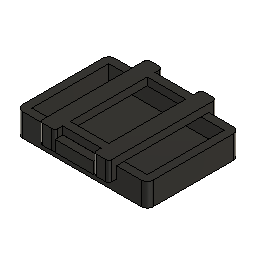
IRreceiverMount (Autodesk Fusion 360 design; units mm, degrees)
Autodesk Fusion 360 part; units mm, degrees
sketch "Sketch1" plane through (0, 0, 0) normal (0, 0, 1) x (1, 0, 0)
  line L0 (0, 0) -> (23.8125, 0)
  line L1 (23.8125, 0) -> (23.8125, 15.875)
  line L2 (23.8125, 15.875) -> (0, 15.875)
  line L3 (0, 15.875) -> (0, 0)
  line L4 (-0.3175, -1.5875) -> (24.13, -1.5875)
  line L5 (25.4, -0.3175) -> (25.4, 16.1925)
  line L6 (24.13, 17.4625) -> (-0.3175, 17.4625)
  line L7 (-1.5875, 16.1925) -> (-1.5875, -0.3175)
  arc A0 (-0.3175, 17.4625) -> (-1.5875, 16.1925) centre (-0.3175, 16.1925) ccw
  arc A1 (-1.5875, -0.3175) -> (-0.3175, -1.5875) centre (-0.3175, -0.3175) ccw
  arc A2 (25.4, 16.1925) -> (24.13, 17.4625) centre (24.13, 16.1925) ccw
  arc A3 (24.13, -1.5875) -> (25.4, -0.3175) centre (24.13, -0.3175) ccw
  dimension "d1" = 23.8125
  dimension "d2" = 15.875
  dimension "d4" = 1.27
  constraint coincident L0.start L3.end
  constraint horizontal L0
  constraint perpendicular L0 L1
  constraint perpendicular L1 L2
  constraint perpendicular L0 L3
  constraint tangent L6 A0
  constraint tangent L7 A0
  constraint tangent L4 A1
  constraint tangent L7 A1
  constraint equal A0 A1
  constraint tangent L5 A2
  constraint tangent L6 A2
  constraint equal A0 A2
  constraint tangent L4 A3
  constraint tangent L5 A3
  constraint equal A0 A3
  measures "d1" distance of L0.start L0.end
  measures "d2" distance of L0.end L1.end
  measures "d4" radius of A0
extrude "Extrude1" add sketch "Sketch1" along normal blind 1.5875 contours L0 L1 L2 L3 makes body 1
extrude "Extrude2" add sketch "Sketch1" along normal blind 4.7625 bodies 1
sketch "Sketch2" plane through (0, 0, 4.7625) normal (0, 0, 1) x (-1, 0, 0)
  line L0 (0, 0) -> (0, -15.875)
  line L1 (0, -15.875) -> (-23.8125, -15.875)
  line L2 (-23.8125, -15.875) -> (-23.8125, 0)
  line L3 (-23.8125, 0) -> (0, 0)
  arc A0 (-24.13, 1.5875) -> (-25.4, 0.3175) centre (-24.13, 0.3175) ccw
  line L4 (-25.4, 0.3175) -> (-25.4, -16.1925)
  arc A1 (-25.4, -16.1925) -> (-24.13, -17.4625) centre (-24.13, -16.1925) ccw
  line L5 (-24.13, -17.4625) -> (0.3175, -17.4625)
  arc A2 (0.3175, -17.4625) -> (1.5875, -16.1925) centre (0.3175, -16.1925) ccw
  line L6 (1.5875, -16.1925) -> (1.5875, 0.3175)
  arc A3 (1.5875, 0.3175) -> (0.3175, 1.5875) centre (0.3175, 0.3175) ccw
  line L7 (0.3175, 1.5875) -> (-24.13, 1.5875)
  line L8 (1.5875, -7.9375) -> (-25.4, -7.9375)
  line L9 (1.5875, -7.9375) -> (-4.7625, -7.9375)
  line L10 (-4.7625, -7.9375) -> (-7.9375, -7.9375)
  line L11 (-25.4, -7.9375) -> (-19.05, -7.9375)
  line L12 (-19.05, -7.9375) -> (-15.875, -7.9375)
  line L13 (-7.9375, -7.9375) -> (-7.9375, 1.5875)
  line L14 (-7.9375, -7.9375) -> (-7.9375, -17.4625)
  line L15 (-7.9375, -17.4625) -> (-4.7625, -17.4625)
  line L16 (-4.7625, -17.4625) -> (-4.7625, 1.5875)
  line L17 (-4.7625, 1.5875) -> (-7.9375, 1.5875)
  line L18 (-15.875, -7.9375) -> (-15.875, -17.4625)
  line L19 (-19.05, -7.9375) -> (-19.05, -17.4625)
  line L20 (-15.875, -17.4625) -> (-19.05, -17.4625)
  line L21 (-19.05, -7.9375) -> (-19.05, 1.5875)
  line L22 (-19.05, 1.5875) -> (-15.875, 1.5875)
  line L23 (-15.875, -7.9375) -> (-15.875, 1.5875)
  line L24 (-7.9375, -15.875) -> (-15.875, -15.875)
  line L25 (-15.875, -17.4625) -> (-7.9375, -17.4625)
  line L26 (-7.9375, 1.5875) -> (-15.875, 1.5875)
  line L27 (-15.875, 0) -> (-7.9375, 0)
  line L28 (-4.7625, 1.5875) -> (-4.7625, 2.54)
  line L29 (-5.3975, 3.175) -> (-7.3025, 3.175)
  line L30 (-7.9375, 2.54) -> (-7.9375, 1.5875)
  line L31 (-15.875, 1.5875) -> (-15.875, 2.54)
  line L32 (-16.51, 3.175) -> (-18.415, 3.175)
  line L33 (-19.05, 2.54) -> (-19.05, 1.5875)
  line L34 (-19.05, -17.4625) -> (-19.05, -18.415)
  line L35 (-18.415, -19.05) -> (-16.51, -19.05)
  line L36 (-15.875, -18.415) -> (-15.875, -17.4625)
  line L37 (-7.9375, -17.4625) -> (-7.9375, -18.415)
  line L38 (-7.3025, -19.05) -> (-5.3975, -19.05)
  line L39 (-4.7625, -18.415) -> (-4.7625, -17.4625)
  arc A4 (-5.3975, -19.05) -> (-4.7625, -18.415) centre (-5.3975, -18.415) ccw
  arc A5 (-7.9375, -18.415) -> (-7.3025, -19.05) centre (-7.3025, -18.415) ccw
  arc A6 (-16.51, -19.05) -> (-15.875, -18.415) centre (-16.51, -18.415) ccw
  arc A7 (-19.05, -18.415) -> (-18.415, -19.05) centre (-18.415, -18.415) ccw
  arc A8 (-4.7625, 2.54) -> (-5.3975, 3.175) centre (-5.3975, 2.54) ccw
  arc A9 (-7.3025, 3.175) -> (-7.9375, 2.54) centre (-7.3025, 2.54) ccw
  arc A10 (-15.875, 2.54) -> (-16.51, 3.175) centre (-16.51, 2.54) ccw
  arc A11 (-18.415, 3.175) -> (-19.05, 2.54) centre (-18.415, 2.54) ccw
  line L40 (-6.35, 1.5875) -> (-6.35, 1.6129)
  line L41 (-6.35, 1.6129) -> (-7.9375, 1.6129)
  line L42 (-6.35, 1.6129) -> (-4.7625, 1.6129)
  line L43 (-17.4625, 1.5875) -> (-17.4625, 1.6129)
  line L44 (-17.4625, 1.6129) -> (-19.05, 1.6129)
  line L45 (-17.4625, 1.6129) -> (-15.875, 1.6129)
  line L46 (-17.4625, -17.4625) -> (-17.4625, -17.4879)
  line L47 (-17.4625, -17.4879) -> (-19.05, -17.4879)
  line L48 (-17.4625, -17.4879) -> (-15.875, -17.4879)
  line L49 (-6.35, -17.4625) -> (-6.35, -17.4879)
  line L50 (-6.35, -17.4879) -> (-7.9375, -17.4879)
  line L51 (-6.35, -17.4879) -> (-4.7625, -17.4879)
  point P0 (-4.7625, 3.175)
  point P1 (-15.875, 3.175)
  point P2 (-19.05, -19.05)
  point P3 (-7.9375, -19.05)
  dimension "d9" = 6.35
  dimension "d10" = 3.175
  dimension "d11" = 6.35
  dimension "d12" = 3.175
  dimension "d13" = 3.175
  dimension "d14" = 3.175
  dimension "d15" = 1.5875
  dimension "d16" = 1.5875
  dimension "d17" = 1.5875
  dimension "d18" = 1.5875
  dimension "d19" = 0.635
  dimension "d22" = 0.0254
  dimension "d23" = 0.0254
  dimension "d24" = 0.0254
  dimension "d25" = 0.0254
  constraint midpoint L6 L8.start
  constraint midpoint L4 L8.end
  constraint coincident L8 L9.end
  constraint perpendicular L0 L10
  constraint perpendicular L2 L11
  constraint perpendicular L2 L12
  constraint coincident L7 L13.end
  constraint perpendicular L7 L13
  constraint coincident L5 L14.end
  constraint perpendicular L5 L14
  constraint coincident L5 L15.end
  constraint coincident L7 L16.end
  constraint perpendicular L7 L16
  constraint coincident L5 L18.end
  constraint perpendicular L5 L18
  constraint coincident L5 L19.end
  constraint perpendicular L5 L19
  constraint coincident L7 L21.end
  constraint perpendicular L7 L21
  constraint coincident L7 L22.end
  constraint coincident L14 L24.start
  constraint coincident L1 L24.start
  constraint coincident L18 L24.end
  constraint coincident L1 L24.end
  constraint coincident L23 L27.start
  constraint coincident L3 L27.start
  constraint coincident L13 L27.end
  constraint coincident L3 L27.end
  constraint perpendicular L17 L28
  constraint perpendicular L13 L29
  constraint perpendicular L26 L30
  constraint perpendicular L26 L31
  constraint perpendicular L21 L32
  constraint perpendicular L22 L33
  constraint perpendicular L20 L34
  constraint perpendicular L18 L35
  constraint perpendicular L25 L36
  constraint perpendicular L25 L37
  constraint perpendicular L16 L38
  constraint perpendicular L15 L39
  constraint tangent L38 A4
  constraint tangent L39 A4
  constraint coincident P3 L38
  constraint coincident P3 L37
  constraint tangent L38 A5
  constraint tangent L37 A5
  constraint equal A4 A5
  constraint tangent L36 A6
  constraint tangent L35 A6
  constraint equal A4 A6
  constraint coincident P2 L34
  constraint coincident P2 L35
  constraint tangent L34 A7
  constraint tangent L35 A7
  constraint equal A4 A7
  constraint coincident P0 L28
  constraint coincident P0 L29
  constraint tangent L28 A8
  constraint tangent L29 A8
  constraint equal A4 A8
  constraint tangent L29 A9
  constraint tangent L30 A9
  constraint equal A4 A9
  constraint coincident P1 L31
  constraint coincident P1 L32
  constraint tangent L31 A10
  constraint tangent L32 A10
  constraint equal A4 A10
  constraint tangent L32 A11
  constraint tangent L33 A11
  constraint equal A4 A11
  constraint midpoint L17 L40.start
  constraint perpendicular L17 L40
  constraint coincident L30 L41.end
  constraint perpendicular L30 L41
  constraint coincident L28 L42.end
  constraint perpendicular L28 L42
  constraint midpoint L22 L43.start
  constraint perpendicular L22 L43
  constraint coincident L33 L44.end
  constraint perpendicular L33 L44
  constraint coincident L31 L45.end
  constraint perpendicular L31 L45
  constraint midpoint L20 L46.start
  constraint perpendicular L20 L46
  constraint coincident L34 L47.end
  constraint perpendicular L34 L47
  constraint perpendicular L18 L48
  constraint midpoint L15 L49.start
  constraint perpendicular L15 L49
  constraint perpendicular L14 L50
  constraint coincident L39 L51.end
  constraint perpendicular L39 L51
  measures "d9" distance of L8.start L9.end
  measures "d10" distance of L9.end L10.end
  measures "d11" distance of L8.end L11.end
  measures "d12" distance of L11.end L12.end
  measures "d13" distance of L14.end L15.end
  measures "d14" distance of L21.end L22.end
  measures "d15" distance of L16.end P0
  measures "d16" distance of L22.end P1
  measures "d17" distance of L19.end P2
  measures "d18" distance of L14.end P3
  measures "d19" radius of A4
  measures "d22" distance of L40.start L40.end
  measures "d23" distance of L43.start L43.end
  measures "d24" distance of L46.start L46.end
  measures "d25" distance of L49.start L49.end
extrude "Extrude3" add sketch "Sketch2" along normal blind 1.5875 separate body contours L3 L8 L10 L13 L16 | L3 L7 L13 L16 L17 | L1 L8 L10 L14 L16 | L3 L7 L13 L23 L26 L27 | L7 L17 L28 L40 L42 | L1 L5 L14 L15 L16 | L3 L8 L12 L21 L23 | L3 L7 L21 L22 L23 | L7 L17 L30 L40 L41 | L28 L29 L30 A8 A9 L41 L42 | L1 L5 L14 L18 L24 L25 | L5 L15 L39 L49 L51 | L1 L8 L12 L18 L19 | L7 L22 L31 L43 L45 | L1 L5 L18 L19 L20 | L5 L15 L37 L49 L50 | L37 L38 L39 A4 A5 L50 L51 | L7 L22 L33 L43 L44 | L31 L32 L33 A10 A11 L44 L45 | L5 L20 L36 L46 L48 | L5 L20 L34 L46 L47 | L34 L35 L36 A6 A7 L47 L48 makes body 2
extrude "Extrude4" add sketch "Sketch2" against normal blind 2.3813 contours L28 L29 L30 A8 A9 L41 L42 | L37 L38 L39 A4 A5 L50 L51 | L31 L32 L33 A10 A11 L44 L45 | L34 L35 L36 A6 A7 L47 L48 bodies 2
sketch "Sketch3" plane through (0, -1.5875, 0) normal (0, -1, 0) x (1, 0, 0)
  line L0 (-0.3175, 0) -> (24.13, 0)
  line L1 (24.13, 0) -> (24.13, 4.7625)
  line L2 (24.13, 4.7625) -> (-0.3175, 4.7625)
  line L3 (-0.3175, 4.7625) -> (-0.3175, 0)
  line L4 (11.9062, 4.7625) -> (15.8432, 4.7625)
  line L5 (15.8432, 4.7625) -> (15.8432, 2.3813)
  line L6 (15.8432, 2.3813) -> (7.9692, 2.3813)
  line L7 (7.9692, 2.3813) -> (7.9692, 4.7625)
  line L8 (7.9692, 4.7625) -> (11.9062, 4.7625)
  line L9 (15.8178, 2.4066) -> (7.9946, 2.4066)
  line L10 (7.9946, 2.4066) -> (7.9946, 4.7371)
  line L11 (7.9946, 4.7371) -> (11.9062, 4.7371)
  line L12 (11.9062, 4.7371) -> (15.8178, 4.7371)
  line L13 (15.8178, 4.7371) -> (15.8178, 2.4066)
  dimension "d28" = 3.937
  dimension "d29" = 2.3813
  dimension "d30" = 7.874
  dimension "d31" = 0.0254
  constraint midpoint L2 L4.start
  constraint parallel L2 L4
  constraint perpendicular L4 L5
  constraint perpendicular L5 L6
  constraint coincident L2 L7.end
  constraint perpendicular L2 L7
  measures "d28" distance of L4.start L4.end
  measures "d29" distance of L4.end L5.end
  measures "d30" distance of L5.end L6.end
extrude "Extrude5" add sketch "Sketch3" along normal blind 1.5875 contours L9 L10 L11 L12 L13 bodies 1
sketch "Sketch4" plane through (0, 17.4625, 0) normal (0, 1, 0) x (-1, 0, 0)
  line L0 (-24.13, 0) -> (0.3175, 0)
  line L1 (0.3175, 0) -> (0.3175, 4.7625)
  line L2 (0.3175, 4.7625) -> (-24.13, 4.7625)
  line L3 (-24.13, 4.7625) -> (-24.13, 0)
  line L4 (-11.9063, 4.7625) -> (-7.9693, 4.7625)
  line L5 (-7.9693, 4.7625) -> (-7.9693, 2.3813)
  line L6 (-7.9693, 2.3813) -> (-15.8433, 2.3813)
  line L7 (-15.8433, 2.3813) -> (-15.8433, 4.7625)
  line L8 (-11.9063, 4.7625) -> (-15.8433, 4.7625)
  line L9 (-7.9947, 2.4066) -> (-15.8179, 2.4066)
  line L10 (-15.8179, 2.4066) -> (-15.8179, 4.7371)
  line L11 (-11.9063, 4.7371) -> (-15.8179, 4.7371)
  line L12 (-11.9063, 4.7371) -> (-7.9947, 4.7371)
  line L13 (-7.9947, 4.7371) -> (-7.9947, 2.4066)
  dimension "d34" = 3.937
  dimension "d35" = 2.3813
  dimension "d36" = 7.874
  dimension "d37" = 0.0254
  constraint midpoint L2 L4.start
  constraint parallel L2 L4
  constraint perpendicular L4 L5
  constraint perpendicular L5 L6
  constraint coincident L2 L7.end
  constraint perpendicular L2 L7
  measures "d34" distance of L4.start L4.end
  measures "d35" distance of L4.end L5.end
  measures "d36" distance of L5.end L6.end
extrude "Extrude6" add sketch "Sketch4" along normal blind 1.5875 contours L9 L10 L11 L12 L13 bodies 1
equation "d1 = ( 15 / 16 ) * 1 in"
equation "d2 = ( 5 / 8 ) * 1 in"
equation "d5 = ( 1 / 16 ) * 1 in"
equation "d7 = ( 3 / 16 ) * 1 in"
equation "d15 = ( 1 / 16 ) * 1 in"
equation "d16 = ( 1 / 16 ) * 1 in"
equation "d17 = ( 1 / 16 ) * 1 in"
equation "d18 = ( 1 / 16 ) * 1 in"
equation "d20 = ( 1 / 16 ) * 1 in"
equation "d26 = ( -3 / 32 ) * 1 in"
equation "d29 = ( 3 / 32 ) * 1 in"
equation "d32 = ( 1 / 16 ) * 1 in"
equation "d35 = ( 3 / 32 ) * 1 in"
equation "d38 = ( 1 / 16 ) * 1 in"
named bodies: "IRmount", "IRcover"
